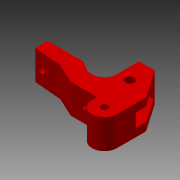
# Autodesk Inventor part: exLever
Saved by Autodesk Inventor 2013 (Build 170138000, 138)
## iProperties
Created: 2015-01-15
Part Number: exLever
Material: Generic
Document SubType Name: Modeling
Designer: dzban
Density: 1 g/cm^3
Author: dzban
Autodesk Inventor part; units mm, degrees
ref_plane "YZ Plane" through (0, 0, 0) normal (1, 0, 0) x (0, 1, 0)
ref_plane "XZ Plane" through (0, 0, 0) normal (0, 1, 0) x (-1, 0, 0)
ref_plane "XY Plane" through (0, 0, 0) normal (0, 0, 1) x (1, 0, 0)
sketch "Sketch1" plane through (0, 0, 0) normal (0, 0, 1) x (1, 0, 0)
  circle A0 centre (-4.7, 16.0016) radius 2
  circle A1 centre (0, 0) radius 1.5
  arc A2 (-18.6289, 10.6759) -> (-9.9, 16.8048) centre (-15.5, 15.5) ccw
  line L0 (-18.6289, 10.6759) -> (-22.3356, 12.8273)
  line L1 (-22.3356, 12.8273) -> (-38, 12.8273)
  line L2 (-38, 12.8273) -> (-38, 7.3273)
  line L3 (-38, 7.3273) -> (-25.7483, 6.2554)
  line L4 (-25.7483, 6.2554) -> (-17.1702, 2.2554)
  line L5 (-17.1702, 2.2554) -> (-5.4202, 2.2554)
  line L6 (-5.4202, 2.2554) -> (-5.4202, 0.9336)
  arc A3 (-5.4202, 0.9336) -> (5.5, 0) centre (0, 0) ccw
  line L7 (5.5, 0) -> (5.5, 12.2919)
  arc A4 (5.5, 12.2919) -> (5.147, 13.4266) centre (3.5, 12.2919) ccw
  line L8 (5.147, 13.4266) -> (-2.9642, 25.2)
  line L9 (-2.9642, 25.2) -> (-9.9, 25.2)
  line L10 (-9.9, 25.2) -> (-9.9, 16.8048)
  constraints: 22 end point, 6 point on circle, 5 centre point
extrude "Extrusion1" add sketch "Sketch1" along normal blind 3.5
sketch "Sketch4" plane through (0, 0, 3.5) normal (0, 0, 1) x (1, 0, 0)
  circle A0 centre (0, 0) radius 1.5 projected
  circle A1 centre (0, 0) radius 1.5
  line L0 (-36.75, 12.8273) -> (-36.75, 11.8273)
  line L1 (-38, 12.8273) -> (-36.75, 12.8273)
  line L2 (-38, 7.3273) -> (-38, 12.8273)
  line L3 (-25.7483, 6.2554) -> (-38, 7.3273)
  line L4 (-17.1702, 2.2554) -> (-25.7483, 6.2554)
  line L5 (-5.4202, 2.2554) -> (-17.1702, 2.2554)
  line L6 (-5.4202, 0.9336) -> (-5.4202, 2.2554)
  arc A2 (-5.4202, 0.9336) -> (5.5, 0) centre (0, 0) ccw
  line L7 (5.5, 8.5016) -> (5.5, 0)
  line L8 (5.5, 8.5016) -> (-4.7, 8.5016)
  arc A3 (-10.9959, 11.9258) -> (-4.7, 8.5016) centre (-4.7, 16.0016) ccw
  arc A4 (-18.6289, 10.6759) -> (-10.9959, 11.9258) centre (-15.5, 15.5) ccw
  line L9 (-22.3356, 12.8273) -> (-18.6289, 10.6759)
  line L10 (-33.25, 12.8273) -> (-22.3356, 12.8273)
  line L11 (-33.25, 12.8273) -> (-33.25, 11.8273)
  line L12 (-33.25, 11.8273) -> (-36.75, 11.8273)
  line L13 (-1.6066, 23.2295) -> (-4.7, 23.5016)
  line L14 (-2.9642, 25.2) -> (-1.6066, 23.2295)
  line L15 (-9.9, 25.2) -> (-2.9642, 25.2)
  line L16 (-9.9, 23.5016) -> (-9.9, 25.2)
  line L17 (-4.7, 23.5016) -> (-9.9, 23.5016)
  constraints: 36 end point, 6 point on circle, 4 centre point
extrude "Extrusion2" add sketch "Sketch4" against normal blind 9.5
sketch "Sketch5" plane through (0, 0, -6) normal (0, 0, -1) x (-1, 0, 0)
  circle A0 centre (0, 0) radius 1.5 projected
  arc A1 (10.9959, 11.9258) -> (18.6289, 10.6759) centre (15.5, 15.5) ccw projected
  arc A2 (4.7, 8.5016) -> (10.9959, 11.9258) centre (4.7, 16.0016) ccw projected
  line L0 (4.7, 8.5016) -> (-5.5, 8.5016) projected
  line L1 (-5.5, 8.5016) -> (-5.5, 0) projected
  arc A3 (-5.5, 0) -> (5.4202, 0.9336) centre (0, 0) ccw projected
  line L2 (5.4202, 0.9336) -> (5.4202, 2.2554) projected
  line L3 (5.4202, 2.2554) -> (17.1702, 2.2554) projected
  line L4 (17.1702, 2.2554) -> (25.7483, 6.2554) projected
  line L5 (25.7483, 6.2554) -> (38, 7.3273) projected
  line L6 (38, 7.3273) -> (38, 12.8273) projected
  line L7 (38, 12.8273) -> (36.75, 12.8273) projected
  line L8 (36.75, 12.8273) -> (36.75, 11.8273) projected
  line L9 (36.75, 11.8273) -> (33.25, 11.8273) projected
  line L10 (33.25, 11.8273) -> (33.25, 12.8273) projected
  line L11 (33.25, 12.8273) -> (22.3356, 12.8273) projected
  line L12 (22.3356, 12.8273) -> (18.6289, 10.6759) projected
  line L13 (-5.5, 8.5016) -> (4.7, 8.5016) projected
  arc A4 (4.7, 8.5016) -> (10.9959, 11.9258) centre (4.7, 16.0016) ccw projected
  arc A5 (9.9, 16.8048) -> (10.9959, 11.9258) centre (15.5, 15.5) ccw projected
  line L14 (9.9, 23.5016) -> (9.9, 16.8048) projected
  line L15 (9.9, 23.5016) -> (4.7, 23.5016) projected
  line L16 (4.7, 23.5016) -> (1.6066, 23.2295) projected
  line L17 (-5.147, 13.4266) -> (1.6066, 23.2295) projected
  arc A6 (-5.147, 13.4266) -> (-5.5, 12.2919) centre (-3.5, 12.2919) ccw projected
  line L18 (-5.5, 8.5016) -> (-5.5, 12.2919) projected
  circle A7 centre (4.7, 16.0016) radius 2 projected
  line L19 (9.9, 23.5016) -> (9.9, 25.2) projected
  line L20 (9.9, 25.2) -> (2.9642, 25.2) projected
  line L21 (2.9642, 25.2) -> (1.6066, 23.2295) projected
  line L22 (1.6066, 23.2295) -> (4.7, 23.5016) projected
  line L23 (4.7, 23.5016) -> (9.9, 23.5016) projected
  line L24 (36.75, 11.8273) -> (36.75, 12.8273) projected
  line L25 (33.25, 12.8273) -> (36.75, 12.8273) projected
  line L26 (33.25, 12.8273) -> (33.25, 11.8273) projected
  line L27 (33.25, 11.8273) -> (36.75, 11.8273) projected
extrude "Extrusion3" add sketch "Sketch5" along normal blind 3.5
sketch "Sketch6" plane through (0, 0, -9.5) normal (0, 0, -1) x (-1, 0, 0)
  arc A0 (9.9, 16.8048) -> (18.6289, 10.6759) centre (15.5, 15.5) ccw projected
  circle A1 centre (15.5, 15.5) radius 7.5
  dimension "d6" = 15
  constraints: 1 centre point, 1 coincident
  measures "d6" diameter of A1
extrude "Extrusion4" cut sketch "Sketch6" against normal blind 3.5
sketch "Sketch7" plane through (-38, 12.8273, 3.5) normal (0, 1, 0) x (1, 0, 0)
  line L0 (0, 13) -> (15.4924, 13) projected
  line L1 (0, 13) -> (0, 0) projected
  line L2 (1.25, 3.5) -> (1.25, 9.5) projected
  circle A0 centre (3, 6.5) radius 1.75
  circle A1 centre (26.8, 6.5) radius 1.1
  point P0 (38, 3.5)
  dimension "d10" = 3.5
  dimension "d13" = 6.5
  dimension "d14" = 26.8
  dimension "d15" = 2.2
  constraints: 2 centre point, 1 horizontal alignment, 1 tangent
  measures "d10" diameter of A0
  measures "d13" distance from line of L0 A0.centre
  measures "d14" distance from line of A1.centre L1
  measures "d15" diameter of A1
extrude "Extrusion5" cut sketch "Sketch7" against normal blind 12
body "Solid1"
